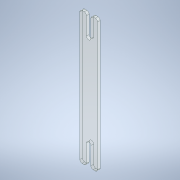
# Autodesk Inventor part: LED_Glass
Saved by Autodesk Inventor 2021 (Build 250183000, 183)
## iProperties
Created: 2020-07-30
Part Number: LED_Glass
Material: Generic
Document SubType Name: Modeling
Designer: CASE-SMALL2
Density: 1 g/cm^3
Appearance: Default
Author: CASE-SMALL2
Autodesk Inventor part; units mm, degrees
ref_plane "YZ Plane" through (0, 0, 0) normal (1, 0, 0) x (0, 1, 0)
ref_plane "XZ Plane" through (0, 0, 0) normal (0, 1, 0) x (-1, 0, 0)
ref_plane "XY Plane" through (0, 0, 0) normal (0, 0, 1) x (1, 0, 0)
sketch "Sketch1" plane through (0, 0, 0) normal (0, 0, 1) x (1, 0, 0)
  line L0 (-10, -75) -> (10, -75)
  line L1 (10, -75) -> (10, 75)
  line L2 (10, 75) -> (-10, 75)
  line L3 (-10, 75) -> (-10, -75)
  line L4 (-10, -75) -> (10, 75) construction
  line L5 (10, -75) -> (-10, 75) construction
  point P0 (0, 0)
  dimension "d0" = 20
  dimension "d1" = 150
  constraints: 12 end point, 2 midpoint, 2 parallel, 1 horizontal, 1 perpendicular
  measures "d0" distance between parallel lines of L1 L3
  measures "d1" distance between parallel lines of L0 L2
extrude "Extrusion1" add sketch "Sketch1" along normal blind 3
sketch "Sketch2" plane through (0, 0, 3) normal (0, 0, 1) x (1, 0, 0)
  line L0 (0, -105) -> (0, 105) construction
  line L1 (-2.5, 50) -> (2.5, 50)
  line L2 (2.5, 50) -> (2.5, 75)
  line L3 (2.5, 75) -> (-2.5, 75)
  line L4 (-2.5, 75) -> (-2.5, 50)
  line L5 (-2.5, 50) -> (2.5, 75) construction
  line L6 (2.5, 50) -> (-2.5, 75) construction
  line L7 (10, 75) -> (-10, 75) construction
  line L8 (-14, 0) -> (14, 0) projected
  line L9 (-2.5, -50) -> (2.5, -50)
  line L10 (2.5, -50) -> (2.5, -75)
  line L11 (2.5, -75) -> (-2.5, -75)
  line L12 (-2.5, -75) -> (-2.5, -50)
  line L13 (-2.5, -50) -> (2.5, -75) construction
  line L14 (2.5, -50) -> (-2.5, -75) construction
  line L15 (10, -75) -> (-10, -75) construction
  point P0 (0, 0)
  point P1 (0, 62.5)
  point P2 (0, 75)
  point P3 (0, -62.5)
  point P4 (0, -75)
  dimension "d4" = 100
  dimension "d5" = 5
  constraints: 26 end point, 8 symmetric about line, 7 midpoint, 2 parallel, 1 horizontal, 1 perpendicular, 1 point on line
  measures "d4" distance between parallel lines of L9 L1
  measures "d5" distance between parallel lines of L2 L4
extrude "Extrusion2" cut sketch "Sketch2" against normal blind 3
fillet "Fillet1" radius 2.5 12 edges at (-2.5, 50, 1.5) (2.5, 50, 1.5) (-2.5, 75, 1.5) (2.5, 75, 1.5) (10, 75, 1.5) (-10, 75, 1.5) (10, -75, 1.5) (-10, -75, 1.5) (-2.5, -75, 1.5) (2.5, -75, 1.5) (-2.5, -50, 1.5) (2.5, -50, 1.5)
sketch "Sketch3" plane through (0, 0, 3) normal (0, 0, 1) x (1, 0, 0)
  arc A0 (2.5, -72.5) -> (5, -75) centre (5, -72.5) ccw projected
  line L0 (5, -75) -> (7.5, -75) projected
  arc A1 (7.5, -75) -> (10, -72.5) centre (7.5, -72.5) ccw projected
  line L1 (10, -72.5) -> (10, 72.5) projected
  arc A2 (10, 72.5) -> (7.5, 75) centre (7.5, 72.5) ccw projected
  line L2 (7.5, 75) -> (5, 75) projected
  arc A3 (5, 75) -> (2.5, 72.5) centre (5, 72.5) ccw projected
  line L3 (2.5, 72.5) -> (2.5, 52.5) projected
  arc A4 (-2.5, 52.5) -> (2.5, 52.5) centre (0, 52.5) ccw projected
  line L4 (-2.5, 52.5) -> (-2.5, 72.5) projected
  arc A5 (-2.5, 72.5) -> (-5, 75) centre (-5, 72.5) ccw projected
  line L5 (-5, 75) -> (-7.5, 75) projected
  arc A6 (-7.5, 75) -> (-10, 72.5) centre (-7.5, 72.5) ccw projected
  line L6 (-10, 72.5) -> (-10, -72.5) projected
  arc A7 (-10, -72.5) -> (-7.5, -75) centre (-7.5, -72.5) ccw projected
  line L7 (-7.5, -75) -> (-5, -75) projected
  arc A8 (-5, -75) -> (-2.5, -72.5) centre (-5, -72.5) ccw projected
  line L8 (-2.5, -72.5) -> (-2.5, -52.5) projected
  arc A9 (2.5, -52.5) -> (-2.5, -52.5) centre (0, -52.5) ccw projected
  line L9 (2.5, -52.5) -> (2.5, -72.5) projected
  point P0 (0, 0)
body "Solid1"
